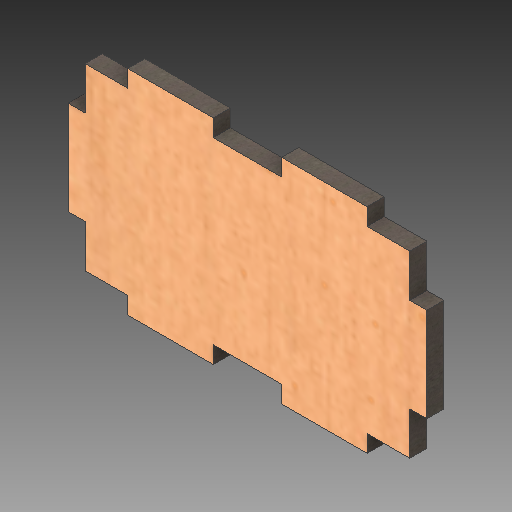
# Autodesk Inventor part: batMain
Saved by Autodesk Inventor 2019 (Build 230136000, 136)
## iProperties
Created: 2020-12-06
Part Number: batMain
Material: Дерево (береза)
Document SubType Name: Modeling
Designer: Professional
Density: 0.55 g/cm^3
Appearance: Береза — натуральный — полированный
Author: Professional
Autodesk Inventor part; units mm, degrees
ref_plane "YZ Plane" through (0, 0, 0) normal (1, 0, 0) x (0, 1, 0)
ref_plane "XZ Plane" through (0, 0, 0) normal (0, 1, 0) x (-1, 0, 0)
ref_plane "XY Plane" through (0, 0, 0) normal (0, 0, 1) x (1, 0, 0)
sketch "Эскиз1" plane through (0, 0, 0) normal (0, 0, 1) x (1, 0, 0)
  line L0 (0, -21) -> (-8, -21)
  line L1 (-8, -21) -> (-8, -25)
  line L2 (-8, -25) -> (-28, -25)
  line L3 (-28, -25) -> (-28, -21)
  line L4 (-28, -21) -> (-38, -21)
  line L5 (-38, -21) -> (-38, -11)
  line L6 (-38, -11) -> (-42, -11)
  line L7 (-42, -11) -> (-42, 0)
  line L8 (-42, 0) -> (0, 0)
  line L9 (0, 21) -> (-8, 21)
  line L10 (-8, 21) -> (-8, 25)
  line L11 (-8, 25) -> (-28, 25)
  line L12 (-28, 25) -> (-28, 21)
  line L13 (-28, 21) -> (-38, 21)
  line L14 (-38, 21) -> (-38, 11)
  line L15 (-38, 11) -> (-42, 11)
  line L16 (-42, 11) -> (-42, 0)
  line L17 (0, -21) -> (0, 21)
  line L18 (0, -21) -> (8, -21)
  line L19 (8, -21) -> (8, -25)
  line L20 (8, -25) -> (28, -25)
  line L21 (28, -25) -> (28, -21)
  line L22 (28, -21) -> (38, -21)
  line L23 (38, -21) -> (38, -11)
  line L24 (38, -11) -> (42, -11)
  line L25 (42, -11) -> (42, 0)
  line L26 (42, 0) -> (0, 0)
  line L27 (0, 21) -> (8, 21)
  line L28 (8, 21) -> (8, 25)
  line L29 (8, 25) -> (28, 25)
  line L30 (28, 25) -> (28, 21)
  line L31 (28, 21) -> (38, 21)
  line L32 (38, 21) -> (38, 11)
  line L33 (38, 11) -> (42, 11)
  line L34 (42, 11) -> (42, 0)
  dimension "d1" = 20
  dimension "d3" = 10
  dimension "d4" = 22
  dimension "d5" = 4
  dimension "d6" = 10
  dimension "d7" = 16
  constraints: 70 end point, 23 symmetric about line, 8 perpendicular, 8 point on line, 1 horizontal, 1 midpoint, 1 vertical
  measures "d1" distance of L1.end L2.end
  measures "d3" distance of L3.end L4.end
  measures "d4" diameter of L6 L8
  measures "d5" distance of L2.end L3.end
  measures "d6" distance of L4.end L5.end
  measures "d7" diameter of L1 L17
extrude "Выдавливание1" add sketch "Эскиз1" along normal blind 4
